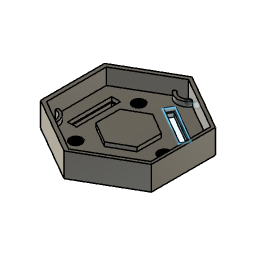
試作品２ v1 (Autodesk Fusion 360 design; units mm, degrees)
Autodesk Fusion 360 part; units mm, degrees
sketch "スケッチ1" plane through (0, 0, 0) normal (0, 0, 1) x (1, 0, 0)
  line L0 (0, 0) -> (69.282, -40)
  line L1 (69.282, -40) -> (138.5641, 0)
  line L2 (138.5641, 0) -> (138.5641, 80)
  line L3 (138.5641, 80) -> (69.282, 120)
  line L4 (69.282, 120) -> (0, 80)
  line L5 (0, 80) -> (0, 0)
  point P0 (69.282, 40)
  constraint coincident L0.start L5.end
extrude "押し出し1" add sketch "スケッチ1" along normal blind 30
sketch "スケッチ2" plane through (0, 0, 30) normal (0, 0, 1) x (-1, 0, 0)
  line L0 (0, -80) -> (0, 0)
  line L1 (0, 0) -> (-69.282, 40)
  line L2 (-69.282, 40) -> (-138.5641, 0)
  line L3 (-138.5641, 0) -> (-138.5641, -80)
  line L4 (-138.5641, -80) -> (-69.282, -120)
  line L5 (-69.282, -120) -> (0, -80)
  line L6 (-96.1204, -54.7555) -> (-70.2816, -69.9987)
  line L7 (-70.2816, -69.9987) -> (-44.1612, -55.2432)
  line L8 (-44.1612, -55.2432) -> (-43.8796, -25.2445)
  line L9 (-43.8796, -25.2445) -> (-69.7184, -10.0013)
  line L10 (-69.7184, -10.0013) -> (-95.8388, -24.7568)
  line L11 (-95.8388, -24.7568) -> (-96.1204, -54.7555)
  line L12 (-134.8251, -77.7188) -> (-69.7472, -114.9996)
  line L13 (-69.7472, -114.9996) -> (-4.922, -77.2808)
  line L14 (-4.922, -77.2808) -> (-5.1749, -2.2812)
  line L15 (-5.1749, -2.2812) -> (-70.2528, 34.9996)
  line L16 (-70.2528, 34.9996) -> (-135.078, -2.7192)
  line L17 (-135.078, -2.7192) -> (-134.8251, -77.7188)
  point P0 (-70, -40)
  point P1 (-70, -40)
  dimension "d3" = 30
  dimension "d4" = 75
  constraint coincident P1 P0
  measures "d3" distance of L6.start P1
  measures "d4" distance of L12.start P1
extrude "押し出し2" cut sketch "スケッチ2" against normal blind 20 contours L12 L13 L14 L15 L16 L17
sketch "スケッチ3" plane through (0, 0, 10) normal (0, 0, 1) x (-1, 0, 0)
  line L0 (-96.1204, -54.7555) -> (-95.8388, -24.7568)
  line L1 (-95.8388, -24.7568) -> (-69.7184, -10.0013)
  line L2 (-69.7184, -10.0013) -> (-43.8796, -25.2445)
  line L3 (-43.8796, -25.2445) -> (-44.1612, -55.2432)
  line L4 (-44.1612, -55.2432) -> (-70.2816, -69.9987)
  line L5 (-70.2816, -69.9987) -> (-96.1204, -54.7555)
  line L6 (-135.078, -2.7192) -> (-134.8251, -77.7188)
  line L7 (-134.8251, -77.7188) -> (-69.7472, -114.9996)
  line L8 (-69.7472, -114.9996) -> (-4.922, -77.2808)
  line L9 (-4.922, -77.2808) -> (-5.1749, -2.2812)
  line L10 (-5.1749, -2.2812) -> (-70.2528, 34.9996)
  line L11 (-70.2528, 34.9996) -> (-135.078, -2.7192)
  line L12 (-112.9332, -60.8656) -> (-118.4398, -70.4033)
  line L13 (-118.4398, -70.4033) -> (-70.8084, -97.9033)
  line L14 (-70.8084, -97.9033) -> (-65.3018, -88.3656)
  line L15 (-65.3018, -88.3656) -> (-112.9332, -60.8656)
  dimension "d7" = 55
  measures "d7" distance of L12.start L14.end
sketch "スケッチ4" plane through (0, 0, 10) normal (0, 0, 1) x (1, 0, 0)
sketch "スケッチ5" plane through (0, 0, 10) normal (0, 0, 1) x (-1, 0, 0)
  line L0 (70, -70) -> (58.7161, -70)
  line L1 (58.7161, -70) -> (58.7161, -15)
  line L2 (58.7161, -15) -> (70, -15)
  line L3 (70, -15) -> (70, -70)
  line L4 (-20.3129, -68.5707) -> (-31.3326, -68.5707)
  line L5 (-31.3326, -68.5707) -> (-31.3326, -13.5707)
  line L6 (-31.3326, -13.5707) -> (-20.3129, -13.5707)
  line L7 (-20.3129, -13.5707) -> (-20.3129, -68.5707)
  dimension "d8" = 55
  dimension "d9" = 55
  constraint horizontal L0
  constraint vertical L1
  constraint horizontal L2
  constraint vertical L3
  constraint horizontal L4
  constraint vertical L5
  constraint horizontal L6
  constraint vertical L7
  measures "d8" distance of L0.start L2.end
  measures "d9" distance of L4.start L6.end
extrude "押し出し3" cut sketch "スケッチ5" against normal blind 5 contours L4 L5 L6 L7
sketch "スケッチ6" plane through (0, 0, 10) normal (0, 0, 1) x (-1, 0, 0)
  line L0 (-30, -15) -> (-21.5271, -15)
  line L1 (-21.5271, -15) -> (-21.5271, -66.9964)
  line L2 (-21.5271, -66.9964) -> (-30, -66.9964)
  line L3 (-30, -66.9964) -> (-30, -15)
  constraint horizontal L0
  constraint vertical L1
  constraint horizontal L2
  constraint vertical L3
extrude "押し出し4" cut sketch "スケッチ6" against normal blind 10
sketch "スケッチ7" plane through (0, 0, 10) normal (0, 0, 1) x (-1, 0, 0)
  line L0 (-117.3805, -6.3384) -> (-69.7491, 21.1616)
  line L1 (-69.7491, 21.1616) -> (-64.1356, 11.4388)
  line L2 (-64.1356, 11.4388) -> (-111.767, -16.0612)
  line L3 (-111.767, -16.0612) -> (-117.3805, -6.3384)
  dimension "d14" = 55
  measures "d14" distance of L0.start L0.end
extrude "押し出し5" cut sketch "スケッチ7" against normal blind 5
sketch "スケッチ8" plane through (0, 0, 0) normal (0, 0, 1) x (1, 0, 0)
  line L0 (111.1427, 14.0503) -> (115.3298, 6.7981)
  line L1 (115.3298, 6.7981) -> (70.488, -19.0913)
  line L2 (70.488, -19.0913) -> (66.301, -11.8391)
  line L3 (66.301, -11.8391) -> (111.1427, 14.0503)
extrude "押し出し6" cut sketch "スケッチ8" along normal blind 5
sketch "スケッチ9" plane through (0, 0, 0) normal (0, 0, 1) x (1, 0, 0)
sketch "スケッチ10" plane through (0, 0, 10) normal (0, 0, 1) x (-1, 0, 0)
  line L0 (-118.4526, -70.4162) -> (-112.7887, -60.6061)
  line L1 (-112.7887, -60.6061) -> (-65.1573, -88.1061)
  line L2 (-65.1573, -88.1061) -> (-70.8212, -97.9162)
  line L3 (-70.8212, -97.9162) -> (-118.4526, -70.4162)
  dimension "d19" = 55
  measures "d19" distance of L0.start L2.end
extrude "押し出し7" cut sketch "スケッチ3" against normal blind 5 contours L12 L13 L14 L15
sketch "スケッチ11" plane through (0, 0, 10) normal (0, 0, 1) x (-1, 0, 0)
  line L0 (-116.3771, -69.7001) -> (-112.376, -62.7699)
  line L1 (-112.376, -62.7699) -> (-67.5978, -88.6226)
  line L2 (-67.5978, -88.6226) -> (-71.5989, -95.5527)
  line L3 (-71.5989, -95.5527) -> (-116.3771, -69.7001)
extrude "押し出し8" cut sketch "スケッチ11" against normal blind 10
hole "穴1" at (45.8897, -1.4293, 10) direction (0, 0, -1) diameter 15 depth 20 tip angle 118
thread "ねじ1" "ISO Metric profile 15.0 M15x1.5 6H" major diameter 15.2033 minor diameter 13.5262 pitch 1.5 angle 60 modelled right hand crest width 0.4068 on face at (46.2636, -8.92, 6.6667) crest through (52.6528, -1.4293, 9.625)
hole "穴2" at (44.5173, 78.5482, 10) direction (0, 0, -1) diameter 15 depth 20 tip angle 118
hole "穴3" at (115.0472, 39.9851, 10) direction (0, 0, -1) diameter 15 depth 20 tip angle 118
thread "ねじ2" "ISO Metric profile 15.0 M15x1.5 6H" major diameter 15.2033 minor diameter 13.5262 pitch 1.5 angle 60 modelled right hand crest width 0.4068 on face at (44.8911, 71.0576, 6.6667) crest through (51.2804, 78.5482, 9.625)
thread "ねじ3" "ISO Metric profile 15.0 M15x1.5 6H" major diameter 15.2033 minor diameter 13.5262 pitch 1.5 angle 60 modelled right hand crest width 0.4068 on face at (115.421, 32.4944, 6.6667) crest through (121.8103, 39.9851, 9.625)
move_body "移動1" bodies 1 to x (1, 0, 0) y (0, 1, 0) z (0, 0, 1) at (-0.7127, 1.4254, 0)
sketch "スケッチ12" plane through (0, 0, 10) normal (0, 0, 1) x (-1, 0, 0)
  spline S0 degree 3 poles (-50.2666, -4.4498) (-50.892, -3.8176) (-51.3863, -3.0681) (-52.0715, -1.4038) (-52.2484, -0.5021) (-52.2506, 1.3396) (-52.0679, 2.2617) (-51.3548, 4.0051) (-50.8241, 4.8065) (-49.7401, 5.9075) (-49.2752, 6.2782) (-48.2611, 6.9064) (-47.7146, 7.1601) (-47.1439, 7.3467) knots 0 0 0 0 0.26677 0.26677 0.539683 0.539683 0.818736 0.818736 1.103927 1.103927 1.281345 1.281345 1.461078 1.461078 1.461078 1.461078
  arc A0 (-43.2102, 7.3467) -> (-47.1439, 7.3467) centre (-45.1771, 0.0039) ccw
  spline S1 degree 3 poles (-43.2102, 7.3467) (-42.2804, 7.0427) (-41.4183, 6.5617) (-39.9451, 5.307) (-39.3432, 4.5513) (-38.4759, 2.8684) (-38.2119, 1.961) (-38.0521, 0.1165) (-38.1501, -0.8021) (-38.5869, -2.1993) (-38.8123, -2.702) (-39.3741, -3.6361) (-39.707, -4.0651) (-40.0875, -4.4498) knots 0 0 0 0 0.293478 0.293478 0.580806 0.580806 0.861983 0.861983 1.137006 1.137006 1.301997 1.301997 1.464671 1.464671 1.464671 1.464671
  arc A1 (-50.2666, -4.4498) -> (-40.0875, -4.4498) centre (-45.1771, 0.0039) ccw
  line L0 (-117.7271, -71.8287) -> (-112.2205, -62.291)
  line L1 (-112.2205, -62.291) -> (-64.5891, -89.791)
  line L2 (-64.5891, -89.791) -> (-70.0957, -99.3287)
  line L3 (-70.0957, -99.3287) -> (-117.7271, -71.8287)
  line L4 (-69.0364, 19.7362) -> (-63.4229, 10.0134)
  line L5 (-63.4229, 10.0134) -> (-111.0543, -17.4866)
  line L6 (-111.0543, -17.4866) -> (-116.6678, -7.7638)
  line L7 (-116.6678, -7.7638) -> (-69.0364, 19.7362)
  line L8 (-30.6199, -69.996) -> (-30.6199, -14.996)
  line L9 (-30.6199, -14.996) -> (-19.6002, -14.996)
  line L10 (-19.6002, -14.996) -> (-19.6002, -69.996)
  line L11 (-19.6002, -69.996) -> (-30.6199, -69.996)
  line L12 (-95.4077, -56.1809) -> (-95.1261, -26.1822)
  line L13 (-95.1261, -26.1822) -> (-69.0057, -11.4267)
  line L14 (-69.0057, -11.4267) -> (-43.1669, -26.6699)
  line L15 (-43.1669, -26.6699) -> (-43.4485, -56.6686)
  line L16 (-43.4485, -56.6686) -> (-69.5689, -71.424)
  line L17 (-69.5689, -71.424) -> (-95.4077, -56.1809)
  line L18 (-134.3653, -4.1446) -> (-134.1124, -79.1441)
  line L19 (-134.1124, -79.1441) -> (-69.0345, -116.4249)
  line L20 (-69.0345, -116.4249) -> (-4.2094, -78.7062)
  line L21 (-4.2094, -78.7062) -> (-4.4622, -3.7066)
  line L22 (-4.4622, -3.7066) -> (-69.5402, 33.5742)
  line L23 (-69.5402, 33.5742) -> (-134.3653, -4.1446)
  spline S2 degree 3 poles (-48.8942, -84.4274) (-49.5195, -83.7951) (-50.0138, -83.0457) (-50.699, -81.3814) (-50.876, -80.4796) (-50.8781, -78.6379) (-50.6954, -77.7158) (-49.9824, -75.9724) (-49.4517, -75.171) (-48.3677, -74.0701) (-47.9027, -73.6993) (-46.8886, -73.0711) (-46.3421, -72.8174) (-45.7714, -72.6308) knots 0 0 0 0 0.26677 0.26677 0.539683 0.539683 0.818736 0.818736 1.103927 1.103927 1.281345 1.281345 1.461078 1.461078 1.461078 1.461078
  arc A2 (-41.8378, -72.6308) -> (-45.7714, -72.6308) centre (-43.8046, -79.9736) ccw
  spline S3 degree 3 poles (-41.8378, -72.6308) (-40.9079, -72.9349) (-40.0458, -73.4158) (-38.5726, -74.6706) (-37.9707, -75.4263) (-37.1034, -77.1092) (-36.8394, -78.0165) (-36.6796, -79.861) (-36.7776, -80.7796) (-37.2145, -82.1769) (-37.4398, -82.6795) (-38.0016, -83.6136) (-38.3345, -84.0427) (-38.715, -84.4274) knots 0 0 0 0 0.293478 0.293478 0.580806 0.580806 0.861983 0.861983 1.137006 1.137006 1.301997 1.301997 1.464671 1.464671 1.464671 1.464671
  arc A3 (-48.8942, -84.4274) -> (-38.715, -84.4274) centre (-43.8046, -79.9736) ccw
  arc A4 (-56.8384, -109.3286) -> (-81.2781, -109.411) centre (-69.0345, -116.4249) ccw
  spline S4 degree 3 poles (-119.4241, -45.8642) (-120.0494, -45.232) (-120.5438, -44.4825) (-121.2289, -42.8182) (-121.4059, -41.9165) (-121.408, -40.0748) (-121.2253, -39.1527) (-120.5123, -37.4092) (-119.9816, -36.6079) (-118.8976, -35.5069) (-118.4326, -35.1362) (-117.4185, -34.508) (-116.872, -34.2543) (-116.3014, -34.0677) knots 0 0 0 0 0.26677 0.26677 0.539683 0.539683 0.818736 0.818736 1.103927 1.103927 1.281345 1.281345 1.461078 1.461078 1.461078 1.461078
  arc A5 (-112.3677, -34.0677) -> (-116.3014, -34.0677) centre (-114.3345, -41.4105) ccw
  spline S5 degree 3 poles (-112.3677, -34.0677) (-111.4379, -34.3717) (-110.5757, -34.8526) (-109.1025, -36.1074) (-108.5007, -36.8631) (-107.6334, -38.546) (-107.3693, -39.4533) (-107.2096, -41.2978) (-107.3075, -42.2165) (-107.7444, -43.6137) (-107.9697, -44.1163) (-108.5315, -45.0505) (-108.8644, -45.4795) (-109.2449, -45.8642) knots 0 0 0 0 0.293478 0.293478 0.580806 0.580806 0.861983 0.861983 1.137006 1.137006 1.301997 1.301997 1.464671 1.464671 1.464671 1.464671
  arc A6 (-119.4241, -45.8642) -> (-109.2449, -45.8642) centre (-114.3345, -41.4105) ccw
  constraint coincident L19 A4.end
  constraint coincident L19.end L20.start
extrude "押し出し9" add sketch "スケッチ12" along normal blind 6 contours L19 L20 A4
sketch "スケッチ13" plane through (0, 0, 16) normal (0, 0, 1) x (-1, 0, 0)
  arc A0 (-56.8384, -109.3286) -> (-81.2781, -109.411) centre (-69.0345, -116.4249) ccw
  line L0 (-81.2781, -109.411) -> (-69.0345, -116.4249)
  line L1 (-69.0345, -116.4249) -> (-56.8384, -109.3286)
  arc A1 (-60.0662, -111.2067) -> (-78.0377, -111.2673) centre (-69.0345, -116.4249) ccw
  constraint coincident L0 A1.end
  constraint coincident A0.centre L0.end
extrude "押し出し10" cut sketch "スケッチ13" against normal blind 10 contours L0 L1 A1
sketch "スケッチ14" plane through (0, 0, 6) normal (0, 0, 1) x (-1, 0, 0)
  arc A0 (-60.0662, -111.2067) -> (-78.0377, -111.2673) centre (-69.0345, -116.4249) ccw
  line L0 (-78.0377, -111.2673) -> (-69.0345, -116.4249)
  line L1 (-69.0345, -116.4249) -> (-60.0662, -111.2067)
  line L2 (-69.0345, -116.4249) -> (-78, -118)
  constraint coincident A0.centre L0.end
sketch "スケッチ15" plane through (0, 0, 10) normal (0, 0, 1) x (-1, 0, 0)
  spline S0 degree 3 poles (-50.2666, -4.4498) (-50.892, -3.8176) (-51.3863, -3.0681) (-52.0715, -1.4038) (-52.2484, -0.5021) (-52.2506, 1.3396) (-52.0679, 2.2617) (-51.3548, 4.0051) (-50.8241, 4.8065) (-49.7401, 5.9075) (-49.2752, 6.2782) (-48.2611, 6.9064) (-47.7146, 7.1601) (-47.1439, 7.3467) knots 0 0 0 0 0.26677 0.26677 0.539683 0.539683 0.818736 0.818736 1.103927 1.103927 1.281345 1.281345 1.461078 1.461078 1.461078 1.461078
  arc A0 (-43.2102, 7.3467) -> (-47.1439, 7.3467) centre (-45.1771, 0.0039) ccw
  spline S1 degree 3 poles (-43.2102, 7.3467) (-42.2804, 7.0427) (-41.4183, 6.5617) (-39.9451, 5.307) (-39.3432, 4.5513) (-38.4759, 2.8684) (-38.2119, 1.961) (-38.0521, 0.1165) (-38.1501, -0.8021) (-38.5869, -2.1993) (-38.8123, -2.702) (-39.3741, -3.6361) (-39.707, -4.0651) (-40.0875, -4.4498) knots 0 0 0 0 0.293478 0.293478 0.580806 0.580806 0.861983 0.861983 1.137006 1.137006 1.301997 1.301997 1.464671 1.464671 1.464671 1.464671
  arc A1 (-50.2666, -4.4498) -> (-40.0875, -4.4498) centre (-45.1771, 0.0039) ccw
  line L0 (-117.7271, -71.8287) -> (-112.2205, -62.291)
  line L1 (-112.2205, -62.291) -> (-64.5891, -89.791)
  line L2 (-64.5891, -89.791) -> (-70.0957, -99.3287)
  line L3 (-70.0957, -99.3287) -> (-117.7271, -71.8287)
  line L4 (-69.0364, 19.7362) -> (-63.4229, 10.0134)
  line L5 (-63.4229, 10.0134) -> (-111.0543, -17.4866)
  line L6 (-111.0543, -17.4866) -> (-116.6678, -7.7638)
  line L7 (-116.6678, -7.7638) -> (-69.0364, 19.7362)
  line L8 (-30.6199, -69.996) -> (-30.6199, -14.996)
  line L9 (-30.6199, -14.996) -> (-19.6002, -14.996)
  line L10 (-19.6002, -14.996) -> (-19.6002, -69.996)
  line L11 (-19.6002, -69.996) -> (-30.6199, -69.996)
  line L12 (-95.4077, -56.1809) -> (-95.1261, -26.1822)
  line L13 (-95.1261, -26.1822) -> (-69.0057, -11.4267)
  line L14 (-69.0057, -11.4267) -> (-43.1669, -26.6699)
  line L15 (-43.1669, -26.6699) -> (-43.4485, -56.6686)
  line L16 (-43.4485, -56.6686) -> (-69.5689, -71.424)
  line L17 (-69.5689, -71.424) -> (-95.4077, -56.1809)
  arc A2 (-56.8384, -109.3286) -> (-81.2781, -109.411) centre (-69.0345, -116.4249) ccw
  line L18 (-56.8384, -109.3286) -> (-4.2094, -78.7062)
  line L19 (-4.2094, -78.7062) -> (-4.4622, -3.7066)
  line L20 (-4.4622, -3.7066) -> (-69.5402, 33.5742)
  line L21 (-69.5402, 33.5742) -> (-134.3653, -4.1446)
  line L22 (-134.3653, -4.1446) -> (-134.1124, -79.1441)
  line L23 (-134.1124, -79.1441) -> (-81.2781, -109.411)
  spline S2 degree 3 poles (-48.8942, -84.4274) (-49.5195, -83.7951) (-50.0138, -83.0457) (-50.699, -81.3814) (-50.876, -80.4796) (-50.8781, -78.6379) (-50.6954, -77.7158) (-49.9824, -75.9724) (-49.4517, -75.171) (-48.3677, -74.0701) (-47.9027, -73.6993) (-46.8886, -73.0711) (-46.3421, -72.8174) (-45.7714, -72.6308) knots 0 0 0 0 0.26677 0.26677 0.539683 0.539683 0.818736 0.818736 1.103927 1.103927 1.281345 1.281345 1.461078 1.461078 1.461078 1.461078
  arc A3 (-41.8378, -72.6308) -> (-45.7714, -72.6308) centre (-43.8046, -79.9736) ccw
  spline S3 degree 3 poles (-41.8378, -72.6308) (-40.9079, -72.9349) (-40.0458, -73.4158) (-38.5726, -74.6706) (-37.9707, -75.4263) (-37.1034, -77.1092) (-36.8394, -78.0165) (-36.6796, -79.861) (-36.7776, -80.7796) (-37.2145, -82.1769) (-37.4398, -82.6795) (-38.0016, -83.6136) (-38.3345, -84.0427) (-38.715, -84.4274) knots 0 0 0 0 0.293478 0.293478 0.580806 0.580806 0.861983 0.861983 1.137006 1.137006 1.301997 1.301997 1.464671 1.464671 1.464671 1.464671
  arc A4 (-48.8942, -84.4274) -> (-38.715, -84.4274) centre (-43.8046, -79.9736) ccw
  spline S4 degree 3 poles (-119.4241, -45.8642) (-120.0494, -45.232) (-120.5438, -44.4825) (-121.2289, -42.8182) (-121.4059, -41.9165) (-121.408, -40.0748) (-121.2253, -39.1527) (-120.5123, -37.4092) (-119.9816, -36.6079) (-118.8976, -35.5069) (-118.4326, -35.1362) (-117.4185, -34.508) (-116.872, -34.2543) (-116.3014, -34.0677) knots 0 0 0 0 0.26677 0.26677 0.539683 0.539683 0.818736 0.818736 1.103927 1.103927 1.281345 1.281345 1.461078 1.461078 1.461078 1.461078
  arc A5 (-112.3677, -34.0677) -> (-116.3014, -34.0677) centre (-114.3345, -41.4105) ccw
  spline S5 degree 3 poles (-112.3677, -34.0677) (-111.4379, -34.3717) (-110.5757, -34.8526) (-109.1025, -36.1074) (-108.5007, -36.8631) (-107.6334, -38.546) (-107.3693, -39.4533) (-107.2096, -41.2978) (-107.3075, -42.2165) (-107.7444, -43.6137) (-107.9697, -44.1163) (-108.5315, -45.0505) (-108.8644, -45.4795) (-109.2449, -45.8642) knots 0 0 0 0 0.293478 0.293478 0.580806 0.580806 0.861983 0.861983 1.137006 1.137006 1.301997 1.301997 1.464671 1.464671 1.464671 1.464671
  arc A6 (-119.4241, -45.8642) -> (-109.2449, -45.8642) centre (-114.3345, -41.4105) ccw
  arc A7 (-16.6296, 3.2637) -> (-4.3358, -17.7286) centre (-4.4622, -3.7066) ccw
  constraint coincident L19.end L20.start
extrude "押し出し11" add sketch "スケッチ15" along normal blind 6 contours L19 L20 A7
sketch "スケッチ16" plane through (0, 0, 16) normal (0, 0, 1) x (-1, 0, 0)
  arc A0 (-16.6296, 3.2637) -> (-4.4149, -17.7291) centre (-4.4622, -3.7066) ccw
  line L0 (-4.4149, -17.7291) -> (-4.4622, -3.7066)
  line L1 (-4.4622, -3.7066) -> (-16.6296, 3.2637)
  arc A1 (-14.007, 1.7612) -> (-4.4125, -14.7065) centre (-4.4622, -3.7066) ccw
  line L2 (-4.4622, -3.7066) -> (-14.007, 1.7612) construction
  line L3 (-4.4622, -3.7066) -> (-4.4125, -14.7065) construction
  dimension "d39" = 11
  dimension "d40" = 120.066
  constraint coincident A0.centre L0.end
  measures "d39" radius of A1
  measures "d40" angle of L2 L3
extrude "押し出し12" cut sketch "スケッチ16" against normal blind 10 contours L0 L1 A1
sketch "スケッチ17" plane through (0, 0, 10) normal (0, 0, 1) x (-1, 0, 0)
  spline S0 degree 3 poles (-119.4241, -45.8642) (-120.0494, -45.232) (-120.5438, -44.4825) (-121.2289, -42.8182) (-121.4059, -41.9165) (-121.408, -40.0748) (-121.2253, -39.1527) (-120.5123, -37.4092) (-119.9816, -36.6079) (-118.8976, -35.5069) (-118.4326, -35.1362) (-117.4185, -34.508) (-116.872, -34.2543) (-116.3014, -34.0677) knots 0 0 0 0 0.26677 0.26677 0.539683 0.539683 0.818736 0.818736 1.103927 1.103927 1.281345 1.281345 1.461078 1.461078 1.461078 1.461078
  arc A0 (-112.3677, -34.0677) -> (-116.3014, -34.0677) centre (-114.3345, -41.4105) ccw
  spline S1 degree 3 poles (-112.3677, -34.0677) (-111.4379, -34.3717) (-110.5757, -34.8526) (-109.1025, -36.1074) (-108.5007, -36.8631) (-107.6334, -38.546) (-107.3693, -39.4533) (-107.2096, -41.2978) (-107.3075, -42.2165) (-107.7444, -43.6137) (-107.9697, -44.1163) (-108.5315, -45.0505) (-108.8644, -45.4795) (-109.2449, -45.8642) knots 0 0 0 0 0.293478 0.293478 0.580806 0.580806 0.861983 0.861983 1.137006 1.137006 1.301997 1.301997 1.464671 1.464671 1.464671 1.464671
  arc A1 (-119.4241, -45.8642) -> (-109.2449, -45.8642) centre (-114.3345, -41.4105) ccw
  spline S2 degree 3 poles (-48.8942, -84.4274) (-49.5195, -83.7951) (-50.0138, -83.0457) (-50.699, -81.3814) (-50.876, -80.4796) (-50.8781, -78.6379) (-50.6954, -77.7158) (-49.9824, -75.9724) (-49.4517, -75.171) (-48.3677, -74.0701) (-47.9027, -73.6993) (-46.8886, -73.0711) (-46.3421, -72.8174) (-45.7714, -72.6308) knots 0 0 0 0 0.26677 0.26677 0.539683 0.539683 0.818736 0.818736 1.103927 1.103927 1.281345 1.281345 1.461078 1.461078 1.461078 1.461078
  arc A2 (-41.8378, -72.6308) -> (-45.7714, -72.6308) centre (-43.8046, -79.9736) ccw
  spline S3 degree 3 poles (-41.8378, -72.6308) (-40.9079, -72.9349) (-40.0458, -73.4158) (-38.5726, -74.6706) (-37.9707, -75.4263) (-37.1034, -77.1092) (-36.8394, -78.0165) (-36.6796, -79.861) (-36.7776, -80.7796) (-37.2145, -82.1769) (-37.4398, -82.6795) (-38.0016, -83.6136) (-38.3345, -84.0427) (-38.715, -84.4274) knots 0 0 0 0 0.293478 0.293478 0.580806 0.580806 0.861983 0.861983 1.137006 1.137006 1.301997 1.301997 1.464671 1.464671 1.464671 1.464671
  arc A3 (-48.8942, -84.4274) -> (-38.715, -84.4274) centre (-43.8046, -79.9736) ccw
  arc A4 (-16.6296, 3.2637) -> (-4.4149, -17.7291) centre (-4.4622, -3.7066) ccw
  line L0 (-16.6296, 3.2637) -> (-69.5402, 33.5742)
  line L1 (-69.5402, 33.5742) -> (-134.3653, -4.1446)
  line L2 (-134.3653, -4.1446) -> (-134.1124, -79.1441)
  line L3 (-134.1124, -79.1441) -> (-81.2781, -109.411)
  arc A5 (-56.8384, -109.3286) -> (-81.2781, -109.411) centre (-69.0345, -116.4249) ccw
  line L4 (-56.8384, -109.3286) -> (-4.2094, -78.7062)
  line L5 (-4.2094, -78.7062) -> (-4.4149, -17.7291)
  line L6 (-95.4077, -56.1809) -> (-95.1261, -26.1822)
  line L7 (-95.1261, -26.1822) -> (-69.0057, -11.4267)
  line L8 (-69.0057, -11.4267) -> (-43.1669, -26.6699)
  line L9 (-43.1669, -26.6699) -> (-43.4485, -56.6686)
  line L10 (-43.4485, -56.6686) -> (-69.5689, -71.424)
  line L11 (-69.5689, -71.424) -> (-95.4077, -56.1809)
  line L12 (-30.6199, -69.996) -> (-30.6199, -14.996)
  line L13 (-30.6199, -14.996) -> (-19.6002, -14.996)
  line L14 (-19.6002, -14.996) -> (-19.6002, -69.996)
  line L15 (-19.6002, -69.996) -> (-30.6199, -69.996)
  line L16 (-69.0364, 19.7362) -> (-63.4229, 10.0134)
  line L17 (-63.4229, 10.0134) -> (-111.0543, -17.4866)
  line L18 (-111.0543, -17.4866) -> (-116.6678, -7.7638)
  line L19 (-116.6678, -7.7638) -> (-69.0364, 19.7362)
  line L20 (-117.7271, -71.8287) -> (-112.2205, -62.291)
  line L21 (-112.2205, -62.291) -> (-64.5891, -89.791)
  line L22 (-64.5891, -89.791) -> (-70.0957, -99.3287)
  line L23 (-70.0957, -99.3287) -> (-117.7271, -71.8287)
  spline S4 degree 3 poles (-50.2666, -4.4498) (-50.892, -3.8176) (-51.3863, -3.0681) (-52.0715, -1.4038) (-52.2484, -0.5021) (-52.2506, 1.3396) (-52.0679, 2.2617) (-51.3548, 4.0051) (-50.8241, 4.8065) (-49.7401, 5.9075) (-49.2752, 6.2782) (-48.2611, 6.9064) (-47.7146, 7.1601) (-47.1439, 7.3467) knots 0 0 0 0 0.26677 0.26677 0.539683 0.539683 0.818736 0.818736 1.103927 1.103927 1.281345 1.281345 1.461078 1.461078 1.461078 1.461078
  arc A6 (-43.2102, 7.3467) -> (-47.1439, 7.3467) centre (-45.1771, 0.0039) ccw
  spline S5 degree 3 poles (-43.2102, 7.3467) (-42.2804, 7.0427) (-41.4183, 6.5617) (-39.9451, 5.307) (-39.3432, 4.5513) (-38.4759, 2.8684) (-38.2119, 1.961) (-38.0521, 0.1165) (-38.1501, -0.8021) (-38.5869, -2.1993) (-38.8123, -2.702) (-39.3741, -3.6361) (-39.707, -4.0651) (-40.0875, -4.4498) knots 0 0 0 0 0.293478 0.293478 0.580806 0.580806 0.861983 0.861983 1.137006 1.137006 1.301997 1.301997 1.464671 1.464671 1.464671 1.464671
  arc A7 (-50.2666, -4.4498) -> (-40.0875, -4.4498) centre (-45.1771, 0.0039) ccw
  arc A8 (-134.3653, -18.1446) -> (-122.2646, 2.8963) centre (-134.3653, -4.1446) ccw
  line L24 (-134.3653, -4.1446) -> (-134.3653, -18.1446) construction
  line L25 (-134.3653, -4.1446) -> (-122.2646, 2.8963) construction
  dimension "d43" = 14
  dimension "d44" = 120.193
  constraint coincident L1.end L2.start
  measures "d43" radius of A8
  measures "d44" angle of L24 L25
extrude "押し出し13" add sketch "スケッチ17" along normal blind 6 contours L1 L2 A8
sketch "スケッチ18" plane through (0, 0, 16) normal (0, 0, 1) x (-1, 0, 0)
  line L0 (-134.3653, -4.1446) -> (-134.3181, -18.1445)
  arc A0 (-134.3181, -18.1445) -> (-122.2646, 2.8963) centre (-134.3653, -4.1446) ccw
  line L1 (-122.2646, 2.8963) -> (-134.3653, -4.1446)
  arc A1 (-134.3282, -15.1445) -> (-124.8576, 1.3875) centre (-134.3653, -4.1446) ccw
  line L2 (-134.3653, -4.1446) -> (-134.3282, -15.1445) construction
  line L3 (-134.3653, -4.1446) -> (-124.8576, 1.3875) construction
  dimension "d47" = 11
  dimension "d48" = 120
  constraint coincident L0.start A0.centre
  measures "d47" radius of A1
  measures "d48" angle of L2 L3
extrude "押し出し14" cut sketch "スケッチ18" against normal blind 10 contours L0 L1 A1
extrude "押し出し15" cut 1 faces at (77.9003, 36.3443, 30) along direction (0, 0, -1) blind 15
